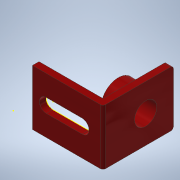
# Autodesk Inventor part: Mancal_Movel
Saved by Autodesk Inventor 2022 (Build 260153000, 153)
## iProperties
Manager: Standard
Created: 2016-02-21
Part Number: Mancal_Movel
Material: SAE 1010/1020
Document SubType Name: Modeling
Designer: Everton
Authority: Rafael Salvador
Manufacturer: Standard
Standards Organization: Custom
Density: 7.86 g/cm^3
Appearance: Steel
Author: Everton
Comments: -
Revision Number: 00
Autodesk Inventor part; units mm, degrees
ref_plane "YZ Plane" through (0, 0, 0) normal (1, 0, 0) x (0, 1, 0)
ref_plane "XZ Plane" through (0, 0, 0) normal (0, 1, 0) x (-1, 0, 0)
ref_plane "XY Plane" through (0, 0, 0) normal (0, 0, 1) x (1, 0, 0)
sketch "Sketch1" plane through (0, 0, 0) normal (0, 0, 1) x (1, 0, 0)
  line L0 (18.6296, 14.5185) -> (69.4296, 14.5185)
  line L1 (69.4296, 14.5185) -> (69.4296, 65.3185)
  line L2 (64.6696, 65.3185) -> (64.6696, 19.2785)
  line L3 (64.6696, 19.2785) -> (18.6296, 19.2785)
  line L4 (18.6296, 19.2785) -> (18.6296, 14.5185)
  line L5 (64.6696, 65.3185) -> (69.4296, 65.3185)
  point P0 (0, 0)
  dimension "d1" = 50.8
  dimension "d2" = 50.8
  dimension "d3" = 4.76
  constraints: 12 end point, 2 vertical, 1 horizontal, 1 other
  measures "d1" distance of L0.start L0.end
  measures "d2" distance of L0.end L1.end
  measures "d3" distance between parallel lines of L1 L2
extrude "Extrusion1" add sketch "Sketch1" along normal blind 40
sketch "Sketch2" plane through (69.4296, 14.5185, 0) normal (1, 0, 0) x (0, 0, -1)
  line L0 (-40, 50.8) -> (0, 0)
  line L1 (-40, 0) -> (0, 50.0964)
  circle A0 centre (-20, 30.8) radius 12.5
  line L2 (0, 50.8) -> (-40, 50.8) projected
  line L3 (0, 0) -> (0, 50.8) projected
  point P0 (0, -14.5185)
  dimension "d6" = 25
  dimension "d7" = 20
  dimension "d8" = 20
  constraints: 4 end point, 1 centre point
  measures "d6" diameter of A0
  measures "d7" distance from line of L2 A0.centre
  measures "d8" distance from line of L3 A0.centre
extrude "Extrusion2" add sketch "Sketch2" against normal blind 19.76 contours A0 L1 L0 | L0 L1 A0 | L1 A0 L0 | L0 A0 L1
sketch "Sketch3" plane through (49.6696, 45.3185, 20) normal (-1, 0, 0) x (0, 0, 1)
  circle A0 centre (0, 0) radius 8
  point P0 (-20, -45.3185)
  dimension "d11" = 16
  constraints: 1 centre point
  measures "d11" diameter of A0
extrude "Extrusion3" cut sketch "Sketch3" against normal blind 19.76
sketch "Sketch4" plane through (18.6296, 14.5185, 0) normal (0, -1, 0) x (1, 0, 0)
  arc A0 (35.8, 15) -> (35.8, 25) centre (35.8, 20) ccw
  arc A1 (10, 25) -> (10, 15) centre (10, 20) ccw
  line L0 (50.8, 0) -> (50.8, 40) projected
  line L1 (0, 0) -> (0, 40) projected
  line L2 (0, 40) -> (50.8, 40) projected
  line L3 (35.8, 25) -> (10, 25)
  line L4 (10, 15) -> (35.8, 15)
  point P0 (-18.6296, 0)
  dimension "d14" = 10
  dimension "d15" = 10
  dimension "d16" = 15
  dimension "d17" = 10
  dimension "d18" = 20
  dimension "d19" = 20
  constraints: 4 end point, 4 point on circle, 2 centre point, 2 tangent
  measures "d14" diameter of A0
  measures "d15" diameter of A1
  measures "d16" distance from line of L0 A0.centre
  measures "d17" distance from line of L1 A1.centre
  measures "d18" distance from line of L2 A0.centre
  measures "d19" distance from line of L2 A1.centre
extrude "Extrusion4" cut sketch "Sketch4" against normal blind 6
fillet "Fillet1" radius 2 1 edges at (69.4296, 14.5185, 20)
fillet "Fillet2" radius 2 2 edges at (67.0496, 65.3185, 40) (67.0496, 65.3185, 0)
sketch "Sketch5" plane through (18.6296, 19.2785, 0) normal (0, 1, 0) x (1, 0, 0)
  arc A0 (35.8, -25) -> (35.8, -15) centre (35.8, -20) ccw projected
  arc A1 (35.8, -25) -> (35.8, -15) centre (35.8, -20) ccw projected
  arc A2 (10, -15) -> (10, -25) centre (10, -20) ccw projected
  line L0 (10, -15) -> (35.8, -15) projected
  line L1 (35.8, -15) -> (10, -15) projected
  line L2 (35.8, -25) -> (10, -25) projected
  point P0 (-18.6296, 0)
equation "\"d19\" = d18"
body "Solid1"
